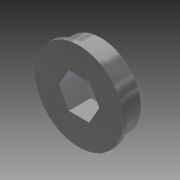
# Autodesk Inventor part: Hex Bearing 1-2 in (FR8ZZ-Hex, am-0279)
Saved by Autodesk Inventor 2014 (Build 180170000, 170)
## iProperties
Created: 2014-01-12
Part Number: Hex Bearing 1-2 in (FR8ZZ-Hex, am-0279)
Material: Steel, Alloy
Document SubType Name: Modeling
Designer: Michael
Density: 7.85 g/cm^3
Appearance: Semi-Polished
Mass: 33.1303 g
Surface Area: 23.8169 cm^2
Volume: 4.22042 cm^3
Author: Michael
Autodesk Inventor part; units mm, degrees
ref_plane "YZ Plane" through (0, 0, 0) normal (1, 0, 0) x (0, 1, 0)
ref_plane "XZ Plane" through (0, 0, 0) normal (0, 1, 0) x (-1, 0, 0)
ref_plane "XY Plane" through (0, 0, 0) normal (0, 0, 1) x (1, 0, 0)
sketch "Sketch1" plane through (0, 0, 0) normal (0, 0, 1) x (1, 0, 0)
  line L0 (3.6662, 6.35) -> (7.3323, 0)
  line L1 (7.3323, 0) -> (3.6662, -6.35)
  line L2 (3.6662, -6.35) -> (-3.6662, -6.35)
  line L3 (-3.6662, -6.35) -> (-7.3323, 0)
  line L4 (-7.3323, 0) -> (-3.6662, 6.35)
  line L5 (-3.6662, 6.35) -> (3.6662, 6.35)
  circle A0 centre (0, 0) radius 14.2875
  dimension "d0" = 12.7
  dimension "d1" = 28.575
  constraints: 12 end point, 2 coincident, 1 centre point, 1 horizontal, 13 other
  measures "d0" distance between parallel lines of L5 L2
  measures "d1" diameter of A0
extrude "Extrusion1" add sketch "Sketch1" along normal blind 6.35
sketch "Sketch2" plane through (0, 0, 6.35) normal (0, 0, 1) x (1, 0, 0)
  circle A0 centre (0, 0) radius 14.2875 projected
  circle A1 centre (0, 0) radius 15.875
  line L0 (-3.6662, 6.35) -> (3.6662, 6.35) projected
  line L1 (3.6662, 6.35) -> (7.3323, 0)
  line L2 (7.3323, 0) -> (3.6662, -6.35)
  line L3 (3.6662, -6.35) -> (-3.6662, -6.35)
  line L4 (-3.6662, -6.35) -> (-7.3323, 0)
  line L5 (-7.3323, 0) -> (-3.6662, 6.35)
  line L6 (-3.6662, 6.35) -> (3.6662, 6.35)
  point P0 (0, 6.35)
  dimension "d4" = 1.5875
  constraints: 12 end point, 2 coincident, 2 midpoint, 1 centre point, 13 other
  measures "d4" radial gap between concentric circles of A1 A0
extrude "Extrusion2" add sketch "Sketch2" along normal blind 1.5875 contours A0 | A1
body "Solid1"
